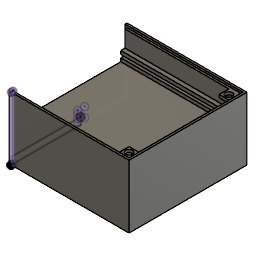
wearable adulto mayor (Autodesk Fusion 360 design; units mm, degrees)
Autodesk Fusion 360 part; units mm, degrees
box "CajaPrimitiva1" add length 85 width 85 height 40 placed x (0, 0, 1) y (1, 0, 0) z (0, 1, 0) at (-50, 0, -50) makes body 1
shell "Vaciado1" thickness 3 removed faces 1 at (6.6667, 40, -21.6667) on bodies 1
box "CajaPrimitiva2" add length 3 width 50 height 20 placed x (0, 0, -1) y (-1, 0, 0) z (0, 1, 0) at (30, 3, -25) bodies 1
box "CajaPrimitiva3" cut length 40 width 85 height -3 placed x (0, 1, 0) y (0, 0, -1) z (-1, 0, 0) at (-50, 0, 35) bodies 1
box "CajaPrimitiva4" add length 50 width 62 height 7 placed x (0, 0, -1) y (-1, 0, 0) z (0, 1, 0) at (15, 3, 25) separate body makes body 2
move_body "Desplazar5" bodies 2 to x (1, 0, 0) y (0, 1, 0) z (0, 0, 1) at (3, 0, 0)
shell "Vaciado2" thickness 5 removed faces 2 at (-44, 5.3333, -8.3333) at (-23.3333, 10, 8.3333) on bodies 2
box "CajaPrimitiva5" cut length 40 width 60 height -5 placed x (0, 0, 1) y (1, 0, 0) z (0, 1, 0) at (-47, 8, -20) bodies 2
sketch "Boceto18" plane through (0, 0, -20) normal (0, 0, 1) x (1, 0, 0)
  line L0 (13, 3) -> (13, 10)
  line L1 (13, 10) -> (-44, 10)
  line L2 (-44, 10) -> (-44, 3)
  line L3 (-44, 3) -> (13, 3)
  line L4 (-44, 5) -> (13, 5)
  arc A0 (13, 5) -> (13, 8) centre (13, 6.5) ccw
  line L5 (13, 8) -> (-44, 8)
  arc A1 (-44, 8) -> (-44, 5) centre (-44, 6.5) ccw
  line L6 (-44, 6.5) -> (13, 6.5) construction
  dimension "d47" = 3
  constraint tangent L4 A0
  constraint tangent A0 L5
  constraint parallel L4 L5
  constraint tangent L5 A1
  constraint tangent L4 A1
  constraint midpoint L0 A0.centre
  constraint perpendicular L0 L6
  constraint midpoint L2 A1.centre
  measures "d47" diameter of A0
extrude "Extruir2" cut sketch "Boceto18" against normal blind 2 contours L0 L2 L4 L5 bodies 2
sketch "Boceto20" plane through (0, 0, 20) normal (0, 0, -1) x (-1, 0, 0)
  line L0 (44, 3) -> (44, 10)
  line L1 (44, 10) -> (-13, 10)
  line L2 (-13, 10) -> (-13, 3)
  line L3 (-13, 3) -> (44, 3)
  line L4 (-13, 5) -> (44, 5)
  arc A0 (44, 5) -> (44, 8) centre (44, 6.5) ccw
  line L5 (44, 8) -> (-13, 8)
  arc A1 (-13, 8) -> (-13, 5) centre (-13, 6.5) ccw
  line L6 (-13, 6.5) -> (44, 6.5) construction
  dimension "d50" = 3
  constraint tangent L4 A0
  constraint tangent A0 L5
  constraint parallel L4 L5
  constraint tangent L5 A1
  constraint tangent L4 A1
  constraint midpoint L0 A0.centre
  constraint perpendicular L0 L6
  constraint midpoint L2 A1.centre
  measures "d50" diameter of A0
extrude "Extruir3" cut sketch "Boceto20" against normal blind 2 contours L0 L2 L4 L5 bodies 2
sketch "Boceto21" plane through (13, 0, 0) normal (-1, 0, 0) x (0, 0, 1)
  line L0 (20, 3) -> (20, 5)
  line L1 (20, 5) -> (22, 5)
  line L2 (22, 5) -> (22, 8)
  line L3 (22, 8) -> (20, 8)
  line L4 (20, 8) -> (20, 10)
  line L5 (20, 10) -> (-20, 10)
  line L6 (-20, 10) -> (-20, 8)
  line L7 (-20, 8) -> (-22, 8)
  line L8 (-22, 8) -> (-22, 5)
  line L9 (-22, 5) -> (-20, 5)
  line L10 (-20, 5) -> (-20, 3)
  line L11 (-20, 3) -> (20, 3)
  line L12 (-22, 5) -> (22, 5)
  arc A0 (22, 5) -> (22, 8) centre (22, 6.5) ccw
  line L13 (22, 8) -> (-22, 8)
  arc A1 (-22, 8) -> (-22, 5) centre (-22, 6.5) ccw
  line L14 (-22, 6.5) -> (22, 6.5) construction
  dimension "d53" = 3
  constraint tangent L12 A0
  constraint tangent A0 L13
  constraint parallel L12 L13
  constraint tangent L13 A1
  constraint tangent L12 A1
  constraint midpoint L2 A0.centre
  constraint perpendicular L2 L14
  constraint midpoint L8 A1.centre
  measures "d53" diameter of A0
extrude "Extruir4" cut sketch "Boceto21" against normal blind 3.5 contours L1 L2 L3 L7 L8 L9 L12 L13 bodies 2
box "CajaPrimitiva1'" add length 9 width 79 height 79 placed x (0, -1, 0) y (-1, 0, 0) z (0, 0, -1) at (32, 30, 32) separate body makes body 3 in component "Component"
shell "Vaciado1'" thickness 1 removed faces 2 at (5.6667, 30, 5.6667) at (-47, 24, 5.6667) on bodies 3 in component "Component"
box "CajaPrimitiva2'" add length 77 width 78 height 1 placed x (0, 0, -1) y (-1, 0, 0) z (0, 1, 0) at (31, 22, 31) bodies 3 in component "Component"
box "CajaPrimitiva3'" cut length 15 width 15 height -2 placed x (0, 0, 1) y (1, 0, 0) z (0, 1, 0) at (16, 23, 16) bodies 3 in component "Component"
box "CajaPrimitiva4'" add length 7 width 78 height 2 placed x (0, 1, 0) y (-1, 0, 0) z (0, 0, 1) at (31, 23, -46) bodies 3 in component "Component"
box "CajaPrimitiva5'" add length 7 width 78 height 2 placed x (0, -1, 0) y (-1, 0, 0) z (0, 0, -1) at (31, 30, 31) bodies 3 in component "Component"
sketch "Boceto31" plane through (0, 0, -44) normal (0, 0, 1) x (1, 0, 0)
  line L0 (31, 30) -> (-47, 30)
  line L1 (-47, 30) -> (-47, 23)
  line L2 (-47, 23) -> (31, 23)
  line L3 (31, 23) -> (31, 30)
  line L4 (-47, 25.5) -> (31, 25.5)
  arc A0 (31, 25.5) -> (31, 27.5) centre (31, 26.5) ccw
  line L5 (31, 27.5) -> (-47, 27.5)
  arc A1 (-47, 27.5) -> (-47, 25.5) centre (-47, 26.5) ccw
  line L6 (-47, 26.5) -> (31, 26.5) construction
  dimension "d82" = 2
  constraint tangent L4 A0
  constraint tangent A0 L5
  constraint parallel L4 L5
  constraint tangent L5 A1
  constraint tangent L4 A1
  constraint midpoint L3 A0.centre
  constraint perpendicular L3 L6
  constraint midpoint L1 A1.centre
  measures "d82" diameter of A0
extrude "Extruir1" cut sketch "Boceto31" against normal blind 2 contours L1 L3 L4 L5 bodies 3 in component "Component"
move_body "Desplazar6" bodies 2 to x (1, 0, 0) y (0, 1, 0) z (0, 0, 1) at (-3, 0, 7)
move_body "Desplazar1" bodies 3 to x (1, 0, 0) y (0, 1, 0) z (0, 0, 1) at (0, 2, 0) in component "Component"
sketch "Boceto37" plane through (0, 0, 29) normal (0, 0, -1) x (-1, 0, 0)
  line L0 (-31, 25) -> (-16, 25)
  line L1 (-16, 25) -> (47, 25)
  line L2 (47, 25) -> (47, 32)
  line L3 (47, 32) -> (-31, 32)
  line L4 (-31, 32) -> (-31, 25)
  line L5 (-32, 27.5) -> (47, 27.5)
  arc A0 (47, 27.5) -> (47, 29.5) centre (47, 28.5) ccw
  line L6 (47, 29.5) -> (-32, 29.5)
  arc A1 (-32, 29.5) -> (-32, 27.5) centre (-32, 28.5) ccw
  line L7 (-32, 28.5) -> (47, 28.5) construction
  constraint tangent L5 A0
  constraint tangent A0 L6
  constraint parallel L5 L6
  constraint tangent L6 A1
  constraint tangent L5 A1
  constraint midpoint L2 A0.centre
  constraint perpendicular L2 L7
extrude "Extruir3'" cut sketch "Boceto37" against normal blind 2 contours L2 L4 L5 L6 bodies 3 in component "Component"
sketch "Boceto38" plane through (31, 0, 0) normal (-1, 0, 0) x (0, 0, 1)
  line L0 (29, 25) -> (29, 27.5)
  line L1 (29, 27.5) -> (31, 27.5)
  line L2 (31, 27.5) -> (31, 29.5)
  line L3 (31, 29.5) -> (29, 29.5)
  line L4 (29, 29.5) -> (29, 32)
  line L5 (29, 32) -> (-44, 32)
  line L6 (-44, 32) -> (-44, 29.5)
  line L7 (-44, 29.5) -> (-46, 29.5)
  line L8 (-46, 29.5) -> (-46, 27.5)
  line L9 (-46, 27.5) -> (-44, 27.5)
  line L10 (-44, 27.5) -> (-44, 25)
  line L11 (-44, 25) -> (16, 25)
  line L12 (16, 25) -> (16, 23)
  line L13 (16, 23) -> (31, 23)
  line L14 (31, 23) -> (31, 25)
  line L15 (31, 25) -> (29, 25)
  line L16 (-46, 27.5) -> (31, 27.5)
  arc A0 (31, 27.5) -> (31, 29.5) centre (31, 28.5) ccw
  line L17 (31, 29.5) -> (-46, 29.5)
  arc A1 (-46, 29.5) -> (-46, 27.5) centre (-46, 28.5) ccw
  line L18 (-46, 28.5) -> (31, 28.5) construction
  constraint tangent L16 A0
  constraint tangent A0 L17
  constraint parallel L16 L17
  constraint tangent L17 A1
  constraint tangent L16 A1
  constraint midpoint L2 A0.centre
  constraint perpendicular L2 L18
  constraint midpoint L8 A1.centre
extrude "Extruir6" cut sketch "Boceto38" against normal blind 2 contours L1 L2 L3 L7 L8 L9 L16 L17 bodies 1
extrude "Extruir4'" cut sketch "Boceto38" against normal blind 2 contours L1 L2 L3 L7 L8 L9 L16 L17 bodies 3 in component "Component"
extrude "Extruir7" add 1 faces at (34, 40, -20.6667) along direction (0, 1, 0) blind 4 on bodies 1 bodies 1
extrude "Extruir8" add 1 faces at (35, 29.3333, -21.6667) along direction (1, 0, 0) blind 3 on bodies 1 bodies 1
extrude "Extruir9" cut 1 faces at (32, 11.1667, 5.3333) along direction (1, 0, 0) blind 3 on bodies 1 bodies 1
sketch "Boceto39" plane through (35, 0, 0) normal (-1, 0, 0) x (0, 0, 1)
  line L0 (-46, 27.5) -> (-46, 29.5)
  line L1 (-46, 29.5) -> (31, 29.5)
  line L2 (31, 29.5) -> (31, 27.5)
  line L3 (31, 27.5) -> (-46, 27.5)
  line L4 (32, 3) -> (32, 44)
  line L5 (32, 44) -> (-47, 44)
  line L6 (-47, 44) -> (-47, 3)
  line L7 (-47, 3) -> (32, 3)
  line L8 (-47, 44) -> (-40, 44)
  line L9 (-40, 44) -> (-40, 42)
  line L10 (-40, 42) -> (-47, 42)
  line L11 (-47, 42) -> (-47, 44)
  line L12 (32, 44) -> (25, 44)
  line L13 (25, 44) -> (25, 42)
  line L14 (25, 42) -> (32, 42)
  line L15 (32, 42) -> (32, 44)
  dimension "d102" = 7
  dimension "d103" = 2
  dimension "d104" = 7
  dimension "d105" = 2
  constraint horizontal L8
  constraint vertical L9
  constraint horizontal L10
  constraint vertical L11
  constraint coincident L5.end L6.start
  constraint horizontal L12
  constraint vertical L13
  constraint horizontal L14
  constraint vertical L15
  constraint coincident L4.end L5.start
  measures "d102" distance of L5.end L8.end
  measures "d103" distance of L5.end L10.end
  measures "d104" distance of L4.end L12.end
  measures "d105" distance of L4.end L14.end
extrude "Extruir10" add sketch "Boceto39" along normal blind 7 contours L4 L5 L12 L13 L14 L15 | L5 L6 L8 L9 L10 L11 bodies 1
sketch "Boceto40" plane through (0, 44, 0) normal (0, 1, 0) x (-1, 0, 0)
  line L0 (-28, 32) -> (47, 32)
  line L1 (47, 32) -> (47, 35)
  line L2 (47, 35) -> (-38, 35)
  line L3 (-38, 35) -> (-38, -50)
  line L4 (-38, -50) -> (47, -50)
  line L5 (47, -50) -> (47, -47)
  line L6 (47, -47) -> (-28, -47)
  line L7 (-28, -47) -> (-28, -40)
  line L8 (-28, -40) -> (-35, -40)
  line L9 (-35, -40) -> (-35, 25)
  line L10 (-35, 25) -> (-28, 25)
  line L11 (-28, 25) -> (-28, 32)
  line L12 (-35, 25) -> (-28, 32)
  circle A0 centre (-31.5, 28.5) radius 2.5
  line L13 (-35, -40) -> (-28, -47)
  circle A1 centre (-31.5, -43.5) radius 2.5
  dimension "d108" = 5
  dimension "d109" = 5
  constraint coincident L9.end L10.start
  constraint coincident L0.start L11.end
  constraint midpoint L12 A0.centre
  constraint coincident L8.end L9.start
  constraint coincident L6.end L7.start
  constraint midpoint L13 A1.centre
  measures "d108" diameter of A0
  measures "d109" diameter of A1
extrude "Extruir11" cut sketch "Boceto40" against normal blind 2 contours L12 A0 | L12 A0 | L13 A1 | L13 A1 bodies 1
sketch "Boceto41" plane through (-47, 0, 0) normal (-1, 0, 0) x (0, 0, 1)
  line L0 (32, 44) -> (32, 3)
  line L1 (32, 3) -> (-47, 3)
  line L2 (-47, 3) -> (-47, 44)
  line L3 (-47, 44) -> (-50, 44)
  line L4 (-50, 44) -> (-50, 0)
  line L5 (-50, 0) -> (35, 0)
  line L6 (35, 0) -> (35, 44)
  line L7 (35, 44) -> (32, 44)
  line L8 (-50, 44) -> (-48.5, 44)
  line L9 (-48.5, 44) -> (-48.5, 0)
  line L10 (-48.5, 0) -> (-50, 0)
  line L11 (-50, 0) -> (-50, 44)
  line L12 (35, 44) -> (33.5, 44)
  line L13 (33.5, 44) -> (33.5, 0)
  line L14 (33.5, 0) -> (35, 0)
  line L15 (35, 0) -> (35, 44)
  dimension "d112" = 1.5
  dimension "d113" = 1.5
  dimension "d114" = 44
  constraint horizontal L8
  constraint vertical L9
  constraint horizontal L10
  constraint vertical L11
  constraint coincident L5 L9.end
  constraint coincident L3.end L4.start
  constraint horizontal L12
  constraint vertical L13
  constraint horizontal L14
  constraint vertical L15
  constraint coincident L6.end L7.start
  measures "d112" distance of L3.end L8.end
  measures "d113" distance of L6.end L12.end
  measures "d114" distance of L6.end L5.end
extrude "Extruir12" add sketch "Boceto41" along normal blind 1.5 contours L5 L6 L7 L12 L13 L14 L15 | L3 L4 L5 L8 L9 L10 L11 bodies 1
sketch "Boceto42" plane through (0, 44, 0) normal (0, 1, 0) x (-1, 0, 0)
  circle A0 centre (-31.5, 28.5) radius 2.5
  circle A1 centre (-31.5, -43.5) radius 2.5
  line L0 (-28, 32) -> (47, 32)
  line L1 (47, 32) -> (47, 33.5)
  line L2 (47, 33.5) -> (48.5, 33.5)
  line L3 (48.5, 33.5) -> (48.5, 35)
  line L4 (48.5, 35) -> (-38, 35)
  line L5 (-38, 35) -> (-38, -50)
  line L6 (-38, -50) -> (48.5, -50)
  line L7 (48.5, -50) -> (48.5, -48.5)
  line L8 (48.5, -48.5) -> (47, -48.5)
  line L9 (47, -48.5) -> (47, -47)
  line L10 (47, -47) -> (-28, -47)
  line L11 (-28, -47) -> (-28, -40)
  line L12 (-28, -40) -> (-35, -40)
  line L13 (-35, -40) -> (-35, 25)
  line L14 (-35, 25) -> (-28, 25)
  line L15 (-28, 25) -> (-28, 32)
  line L16 (47, 33.5) -> (-36.5, 33.5)
  line L17 (-36.5, 33.5) -> (-36.5, -48.5)
  line L18 (-36.5, -48.5) -> (48.5, -48.5)
  dimension "d117" = 83.5
  dimension "d118" = 82
  constraint coincident L1.end L2.start
  constraint perpendicular L5 L16
  constraint perpendicular L6 L17
  constraint coincident L7.end L8.start
  measures "d117" distance of L1.end L16.end
  measures "d118" distance of L16.end L17.end
extrude "Extruir13" add sketch "Boceto42" along normal blind 1.5 contours L2 L3 L4 L5 L6 L7 L8 L16 L17 L18 bodies 1
sketch "Boceto43" plane through (-47, 0, 0) normal (-1, 0, 0) x (0, 0, 1)
  line L0 (33.5, 0) -> (33.5, 44)
  line L1 (33.5, 44) -> (32, 44)
  line L2 (32, 44) -> (32, 3)
  line L3 (32, 3) -> (-47, 3)
  line L4 (-47, 3) -> (-47, 44)
  line L5 (-47, 44) -> (-48.5, 44)
  line L6 (-48.5, 44) -> (-48.5, 0)
  line L7 (-48.5, 0) -> (33.5, 0)
  line L8 (35, 0) -> (35, 45.5)
  line L9 (35, 45.5) -> (33.5, 45.5)
  line L10 (33.5, 45.5) -> (33.5, 0)
  line L11 (33.5, 0) -> (35, 0)
  line L12 (-15, 8) -> (-13, 8)
  line L13 (-13, 8) -> (-13, 10)
  line L14 (-13, 10) -> (-18, 10)
  line L15 (-18, 10) -> (-18, 3)
  line L16 (-18, 3) -> (-13, 3)
  line L17 (-13, 3) -> (-13, 5)
  line L18 (-13, 5) -> (-15, 5)
  line L19 (-15, 5) -> (-15, 8)
  line L20 (35, 0) -> (-15, 0)
  line L21 (-15, 0) -> (-15, 5)
  line L22 (-15, 5) -> (35, 5)
  line L23 (35, 5) -> (35, 0)
  constraint horizontal L20
  constraint vertical L21
  constraint horizontal L22
  constraint vertical L23
  constraint coincident L18.end L19.start
  constraint coincident L8.start L11.end
component "Component" placed x (1, 0, 0) y (0, 1, 0) z (0, 0, 1) at (0, 0, 0)
